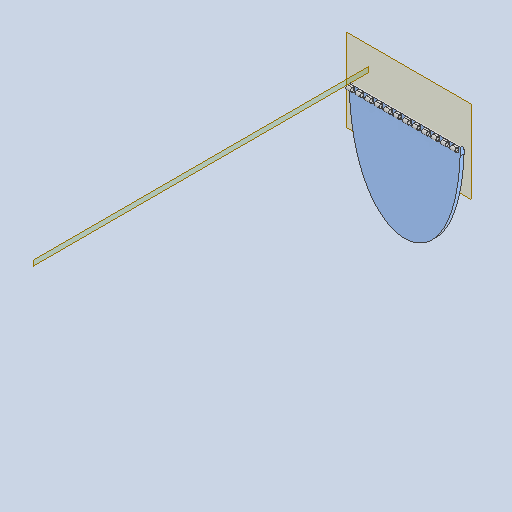
# Autodesk Inventor part: back-flaps-3
Saved by Autodesk Inventor 2023 (Build 270158030, 158C)
## iProperties
Created: 2024-09-10
Part Number: back-flaps-3
Material: Generic
Document SubType Name: Modeling
Designer: Imogen Heard
Density: 1 g/cm^3
Appearance: Default
Author: Imogen Heard
Autodesk Inventor part; units mm, degrees
ref_plane "YZ Plane" through (0, 0, 0) normal (1, 0, 0) x (0, 1, 0)
ref_plane "XZ Plane" through (0, 0, 0) normal (0, 1, 0) x (-1, 0, 0)
ref_plane "XY Plane" through (0, 0, 0) normal (0, 0, 1) x (1, 0, 0)
ref_plane "Work Plane1" through (-701.2547, 0, 0) normal (0, 0, 1) x (1, 0, 0)
sketch "Sketch1" plane through (-701.2547, 0, 0) normal (0, 0, 1) x (1, 0, 0)
  line L0 (557.3903, 26) -> (429.8698, 26) projected
  arc A0 (429.8698, 26) -> (429.8698, 4) centre (429.8698, 15) ccw projected
  line L1 (429.8698, 4) -> (557.3903, 4) projected
  arc A1 (557.3903, 4) -> (557.3903, 26) centre (557.3903, 15) ccw projected
  line L2 (701.2547, 0) -> (1.2547, 0) projected
  line L3 (1.2547, 0) -> (1.2547, 30) projected
  line L4 (1.2547, 30) -> (701.2547, 30) projected
  line L5 (701.2547, 30) -> (701.2547, 0) projected
  line L6 (1.2547, 0) -> (701.2547, 0)
  line L7 (701.2547, 0) -> (701.2547, -50)
  line L8 (701.2547, -50) -> (1.2547, -50)
  line L9 (1.2547, -50) -> (1.2547, 0)
  line L10 (1.2547, -50) -> (31.2547, -700) construction
  line L11 (31.2547, -700) -> (351.2547, -850) construction
  line L12 (351.2547, -850) -> (671.2547, -700) construction
  line L13 (671.2547, -700) -> (701.2547, -50) construction
  spline S0 degree 4 poles (1.2547, -50) (31.2547, -700) (351.2547, -850) (671.2547, -700) (701.2547, -50) knots 1 1 1 1 1 2 2 2 2 2
  dimension "d0" = 50
  dimension "d1" = 850
  dimension "d2" = 700
  dimension "d3" = 30
  dimension "d4" = 30
  dimension "d5" = 350
  dimension "d6" = 350
  constraints: 8 end point, 2 parallel, 1 horizontal, 1 horizontal alignment, 1 perpendicular, 1 vertical alignment, 3 other
  measures "d0" distance between parallel lines of L6 L8
  measures "d1" distance from line of L11.end L2
  measures "d2" distance from line of L2 L10.end
  measures "d3" distance from line of L10.end L3
  measures "d4" distance from line of L12.end L7
  measures "d5" distance from line of L7 L11.end
  measures "d6" distance from line of L9 L11.end
extrude "Extrusion1" add sketch "Sketch1" along normal blind 25 contours L7 L8 L9 L2 | S0 L8
ref_plane "Work Plane2" through (-700, 0, 1930) normal (-1, 0, 0) x (0, 1, 0)
sketch "Sketch3" plane through (-700, -50, 0) normal (-1, 0, 0) x (0, 0, 1)
  circle A0 centre (37.5, 36) radius 12.5
  line L0 (0, 50) -> (25, 50) projected
  line L1 (25, 50) -> (25, 0) projected
  circle A1 centre (37.5, 36) radius 10
  arc A2 (40.5, 23.8653) -> (25, 13.8653) centre (45.3472, -0.6603) ccw
  line L2 (37.5, 48.5) -> (25, 48.5)
  point P0 (12.5, 50)
  point P1 (39.7301, 23.7006)
  point P2 (25, 36)
  point P3 (25, 41.0707)
  dimension "d11" = 12.5
  dimension "d12" = 2.5
  dimension "d13" = 20
  dimension "d14" = 10
  dimension "d15" = 3
  dimension "d16" = 25
  dimension "d17" = 14
  dimension "d18" = 12.5
  constraints: 4 point on circle, 3 centre point, 2 end point, 1 midpoint, 1 perpendicular, 1 point on line, 1 vertical alignment
  measures "d11" distance from line of L1 A1.centre
  measures "d12" radial gap between concentric circles of A0 A1
  measures "d13" diameter of A1
  measures "d14" vertical distance of A2.end A0.start
  measures "d15" horizontal distance of A1.centre A0.start
  measures "d16" radius of A2
  measures "d17" distance from line of L0 A1.centre
  measures "d18" distance from line of L2 A1.centre
extrude "Extrusion2" add sketch "Sketch3" against normal blind 30
fillet "Fillet1" radius 25 1 edges at (-350, 0, 0)
pattern_linear "Rectangular Pattern1" count 12 spacing 60 along (1, 0, 0) of "Extrusion2"
